Autodesk Inventor part; units mm, degrees
(part 3 of 3)
  line L541 (30.6809, 2.8888) -> (31.1045, 2.7392)
  line L542 (31.1045, 2.7392) -> (31.1501, 2.1604)
  line L543 (31.1501, 2.1604) -> (30.7551, 1.9463)
  line L544 (30.7551, 1.9463) -> (30.3579, 1.7492)
  line L545 (30.3579, 1.7492) -> (29.9589, 1.5701)
  line L546 (29.9589, 1.5701) -> (29.5581, 1.4102)
  line L547 (29.5581, 1.4102) -> (29.1557, 1.2717)
  line L548 (29.1557, 1.2717) -> (28.9539, 1.2113)
  line L549 (28.9539, 1.2113) -> (28.8529, 1.1836)
  line L550 (28.8529, 1.1836) -> (28.7518, 1.1577)
  line L551 (28.7518, 1.1577) -> (28.773, 0.3487)
  line L552 (28.773, 0.3487) -> (28.8753, 0.3281)
  line L553 (28.8753, 0.3281) -> (28.9776, 0.3057)
  line L554 (28.9776, 0.3057) -> (29.1823, 0.256)
  line L555 (29.1823, 0.256) -> (29.5914, 0.1387)
  line L556 (29.5914, 0.1387) -> (30, 0)
  line L557 (30, 0) -> (30.4079, -0.158)
  line L558 (30.4079, -0.158) -> (30.8148, -0.3341)
  line L559 (30.8148, -0.3341) -> (31.2205, -0.5271)
  line L560 (31.2205, -0.5271) -> (31.2053, -1.1075)
  line L561 (31.2053, -1.1075) -> (30.7901, -1.2791)
  line L562 (30.7901, -1.2791) -> (30.3745, -1.4336)
  line L563 (30.3745, -1.4336) -> (29.9589, -1.5701)
  line L564 (29.9589, -1.5701) -> (29.5436, -1.6872)
  line L565 (29.5436, -1.6872) -> (29.1289, -1.7829)
  line L566 (29.1289, -1.7829) -> (28.9219, -1.8218)
  line L567 (28.9219, -1.8218) -> (28.8186, -1.8388)
  line L568 (28.8186, -1.8388) -> (28.7153, -1.854)
  line L569 (28.7153, -1.854) -> (28.6518, -2.6609)
  line L570 (28.6518, -2.6609) -> (28.7514, -2.692)
  line L571 (28.7514, -2.692) -> (28.8508, -2.725)
  line L572 (28.8508, -2.725) -> (29.0492, -2.7958)
  line L573 (29.0492, -2.7958) -> (29.4438, -2.9552)
  line L574 (29.4438, -2.9552) -> (29.8357, -3.1359)
  line L575 (29.8357, -3.1359) -> (30.2248, -3.3356)
  line L576 (30.2248, -3.3356) -> (30.6111, -3.5533)
  line L577 (30.6111, -3.5533) -> (30.9943, -3.7877)
  line L578 (30.9943, -3.7877) -> (30.9185, -4.3633)
  line L579 (30.9185, -4.3633) -> (30.4877, -4.4905)
  line L580 (30.4877, -4.4905) -> (30.0582, -4.6008)
  line L581 (30.0582, -4.6008) -> (29.6307, -4.693)
  line L582 (29.6307, -4.693) -> (29.2054, -4.7661)
  line L583 (29.2054, -4.7661) -> (28.7829, -4.8179)
  line L584 (28.7829, -4.8179) -> (28.5731, -4.835)
  line L585 (28.5731, -4.835) -> (28.4685, -4.8411)
  line L586 (28.4685, -4.8411) -> (28.3642, -4.8455)
  line L587 (28.3642, -4.8455) -> (28.2167, -5.6412)
  line L588 (28.2167, -5.6412) -> (28.3125, -5.6826)
  line L589 (28.3125, -5.6826) -> (28.408, -5.7258)
  line L590 (28.408, -5.7258) -> (28.5978, -5.8169)
  line L591 (28.5978, -5.8169) -> (28.9736, -6.0168)
  line L592 (28.9736, -6.0168) -> (29.3444, -6.2373)
  line L593 (29.3444, -6.2373) -> (29.7106, -6.4767)
  line L594 (29.7106, -6.4767) -> (30.072, -6.7335)
  line L595 (30.072, -6.7335) -> (30.4286, -7.0067)
  line L596 (30.4286, -7.0067) -> (30.2931, -7.5713)
  line L597 (30.2931, -7.5713) -> (29.8513, -7.6528)
  line L598 (29.8513, -7.6528) -> (29.4127, -7.7175)
  line L599 (29.4127, -7.7175) -> (28.9778, -7.7646)
  line L600 (28.9778, -7.7646) -> (28.5472, -7.7927)
  line L601 (28.5472, -7.7927) -> (28.1217, -7.8002)
  line L602 (28.1217, -7.8002) -> (27.9111, -7.7952)
  line L603 (27.9111, -7.7952) -> (27.8065, -7.7904)
  line L604 (27.8065, -7.7904) -> (27.7023, -7.7838)
  line L605 (27.7023, -7.7838) -> (27.4725, -8.5597)
  line L606 (27.4725, -8.5597) -> (27.5634, -8.611)
  line L607 (27.5634, -8.611) -> (27.6538, -8.6638)
  line L608 (27.6538, -8.6638) -> (27.8331, -8.7744)
  line L609 (27.8331, -8.7744) -> (28.1859, -9.0124)
  line L610 (28.1859, -9.0124) -> (28.5317, -9.2705)
  line L611 (28.5317, -9.2705) -> (28.8708, -9.5468)
  line L612 (28.8708, -9.5468) -> (29.2034, -9.84)
  line L613 (29.2034, -9.84) -> (29.5295, -10.149)
  line L614 (29.5295, -10.149) -> (29.3357, -10.6963)
  line L615 (29.3357, -10.6963) -> (28.8878, -10.7312)
  line L616 (28.8878, -10.7312) -> (28.4448, -10.7497)
  line L617 (28.4448, -10.7497) -> (28.0074, -10.751)
  line L618 (28.0074, -10.751) -> (27.5762, -10.7341)
  line L619 (27.5762, -10.7341) -> (27.1523, -10.697)
  line L620 (27.1523, -10.697) -> (26.9434, -10.67)
  line L621 (26.9434, -10.67) -> (26.8398, -10.6543)
  line L622 (26.8398, -10.6543) -> (26.7369, -10.6368)
  line L623 (26.7369, -10.6368) -> (26.4272, -11.3845)
  line L624 (26.4272, -11.3845) -> (26.5123, -11.4449)
  line L625 (26.5123, -11.4449) -> (26.5967, -11.507)
  line L626 (26.5967, -11.507) -> (26.7635, -11.6357)
  line L627 (26.7635, -11.6357) -> (27.0895, -11.9092)
  line L628 (27.0895, -11.9092) -> (27.4064, -12.2021)
  line L629 (27.4064, -12.2021) -> (27.7147, -12.5124)
  line L630 (27.7147, -12.5124) -> (28.0148, -12.8387)
  line L631 (28.0148, -12.8387) -> (28.3069, -13.1801)
  line L632 (28.3069, -13.1801) -> (28.057, -13.7041)
  line L633 (28.057, -13.7041) -> (27.6078, -13.692)
  line L634 (27.6078, -13.692) -> (27.1654, -13.6641)
  line L635 (27.1654, -13.6641) -> (26.7302, -13.6197)
  line L636 (26.7302, -13.6197) -> (26.3032, -13.5578)
  line L637 (26.3032, -13.5578) -> (25.8854, -13.4766)
  line L638 (25.8854, -13.4766) -> (25.6805, -13.4279)
  line L639 (25.6805, -13.4279) -> (25.5791, -13.4014)
  line L640 (25.5791, -13.4014) -> (25.4786, -13.3733)
  line L641 (25.4786, -13.3733) -> (25.0925, -14.0845)
  line L642 (25.0925, -14.0845) -> (25.1708, -14.1535)
  line L643 (25.1708, -14.1535) -> (25.2482, -14.2241)
  line L644 (25.2482, -14.2241) -> (25.4006, -14.3694)
  line L645 (25.4006, -14.3694) -> (25.6962, -14.6756)
  line L646 (25.6962, -14.6756) -> (25.9808, -15)
  line L647 (25.9808, -15) -> (26.255, -15.3408)
  line L648 (26.255, -15.3408) -> (26.5194, -15.6967)
  line L649 (26.5194, -15.6967) -> (26.7741, -16.0667)
  line L650 (26.7741, -16.0667) -> (26.4708, -16.5618)
  line L651 (26.4708, -16.5618) -> (26.0254, -16.5028)
  line L652 (26.0254, -16.5028) -> (25.5883, -16.4288)
  line L653 (25.5883, -16.4288) -> (25.1601, -16.3392)
  line L654 (25.1601, -16.3392) -> (24.7419, -16.2329)
  line L655 (24.7419, -16.2329) -> (24.3349, -16.1085)
  line L656 (24.3349, -16.1085) -> (24.1362, -16.0387)
  line L657 (24.1362, -16.0387) -> (24.0382, -16.0018)
  line L658 (24.0382, -16.0018) -> (23.9412, -15.9633)
  line L659 (23.9412, -15.9633) -> (23.4828, -16.6303)
  line L660 (23.4828, -16.6303) -> (23.5534, -16.7071)
  line L661 (23.5534, -16.7071) -> (23.6231, -16.7853)
  line L662 (23.6231, -16.7853) -> (23.7594, -16.9458)
  line L663 (23.7594, -16.9458) -> (24.0214, -17.2812)
  line L664 (24.0214, -17.2812) -> (24.2705, -17.6336)
  line L665 (24.2705, -17.6336) -> (24.5076, -18.0012)
  line L666 (24.5076, -18.0012) -> (24.7333, -18.3827)
  line L667 (24.7333, -18.3827) -> (24.948, -18.7774)
  line L668 (24.948, -18.7774) -> (24.5946, -19.238)
  line L669 (24.5946, -19.238) -> (24.1578, -19.1328)
  line L670 (24.1578, -19.1328) -> (23.7308, -19.0135)
  line L671 (23.7308, -19.0135) -> (23.3144, -18.8796)
  line L672 (23.3144, -18.8796) -> (22.9095, -18.7302)
  line L673 (22.9095, -18.7302) -> (22.5178, -18.5639)
  line L674 (22.5178, -18.5639) -> (22.3275, -18.4738)
  line L675 (22.3275, -18.4738) -> (22.2339, -18.4268)
  line L676 (22.2339, -18.4268) -> (22.1414, -18.3784)
  line L677 (22.1414, -18.3784) -> (21.6158, -18.9938)
  line L678 (21.6158, -18.9938) -> (21.6781, -19.0775)
  line L679 (21.6781, -19.0775) -> (21.7391, -19.1626)
  line L680 (21.7391, -19.1626) -> (21.8579, -19.3365)
  line L681 (21.8579, -19.3365) -> (22.0835, -19.6974)
  line L682 (22.0835, -19.6974) -> (22.2943, -20.0739)
  line L683 (22.2943, -20.0739) -> (22.4917, -20.4643)
  line L684 (22.4917, -20.4643) -> (22.6763, -20.8674)
  line L685 (22.6763, -20.8674) -> (22.8486, -21.2823)
  line L686 (22.8486, -21.2823) -> (22.4489, -21.7034)
  line L687 (22.4489, -21.7034) -> (22.0256, -21.5531)
  line L688 (22.0256, -21.5531) -> (21.6134, -21.3899)
  line L689 (21.6134, -21.3899) -> (21.2132, -21.2132)
  line L690 (21.2132, -21.2132) -> (20.8262, -21.0223)
  line L691 (20.8262, -21.0223) -> (20.454, -20.816)
  line L692 (20.454, -20.816) -> (20.2741, -20.7064)
  line L693 (20.2741, -20.7064) -> (20.1859, -20.6499)
  line L694 (20.1859, -20.6499) -> (20.099, -20.5921)
  line L695 (20.099, -20.5921) -> (19.512, -21.1492)
  line L696 (19.512, -21.1492) -> (19.5652, -21.239)
  line L697 (19.5652, -21.239) -> (19.617, -21.33)
  line L698 (19.617, -21.33) -> (19.717, -21.5154)
  line L699 (19.717, -21.5154) -> (19.9035, -21.8979)
  line L700 (19.9035, -21.8979) -> (20.0739, -22.2943)
  line L701 (20.0739, -22.2943) -> (20.2294, -22.7032)
  line L702 (20.2294, -22.7032) -> (20.3709, -23.1234)
  line L703 (20.3709, -23.1234) -> (20.4988, -23.5541)
  line L704 (20.4988, -23.5541) -> (20.0573, -23.9311)
  line L705 (20.0573, -23.9311) -> (19.652, -23.7374)
  line L706 (19.652, -23.7374) -> (19.2591, -23.5319)
  line L707 (19.2591, -23.5319) -> (18.8796, -23.3144)
  line L708 (18.8796, -23.3144) -> (18.5147, -23.0841)
  line L709 (18.5147, -23.0841) -> (18.1661, -22.84)
  line L710 (18.1661, -22.84) -> (17.9986, -22.7122)
  line L711 (17.9986, -22.7122) -> (17.9169, -22.6468)
  line L712 (17.9169, -22.6468) -> (17.8365, -22.5802)
  line L713 (17.8365, -22.5802) -> (17.1944, -23.0729)
  line L714 (17.1944, -23.0729) -> (17.2379, -23.1678)
  line L715 (17.2379, -23.1678) -> (17.2799, -23.2637)
  line L716 (17.2799, -23.2637) -> (17.36, -23.4585)
  line L717 (17.36, -23.4585) -> (17.5056, -23.8584)
  line L718 (17.5056, -23.8584) -> (17.6336, -24.2705)
  line L719 (17.6336, -24.2705) -> (17.7455, -24.6934)
  line L720 (17.7455, -24.6934) -> (17.8422, -25.1261)
  line L721 (17.8422, -25.1261) -> (17.9245, -25.5677)
  line L722 (17.9245, -25.5677) -> (17.446, -25.8966)
  line L723 (17.446, -25.8966) -> (17.0631, -25.6615)
  line L724 (17.0631, -25.6615) -> (16.6939, -25.4161)
  line L725 (16.6939, -25.4161) -> (16.3392, -25.1601)
  line L726 (16.3392, -25.1601) -> (16.0003, -24.8929)
  line L727 (16.0003, -24.8929) -> (15.6791, -24.6137)
  line L728 (15.6791, -24.6137) -> (15.526, -24.4692)
  line L729 (15.526, -24.4692) -> (15.4515, -24.3955)
  line L730 (15.4515, -24.3955) -> (15.3785, -24.3209)
  line L731 (15.3785, -24.3209) -> (14.6884, -24.7438)
  line L732 (14.6884, -24.7438) -> (14.7218, -24.8427)
  line L733 (14.7218, -24.8427) -> (14.7536, -24.9425)
  line L734 (14.7536, -24.9425) -> (14.8128, -25.1446)
  line L735 (14.8128, -25.1446) -> (14.9158, -25.5575)
  line L736 (14.9158, -25.5575) -> (15, -25.9808)
  line L737 (15, -25.9808) -> (15.0671, -26.413)
  line L738 (15.0671, -26.413) -> (15.1181, -26.8534)
  line L739 (15.1181, -26.8534) -> (15.1537, -27.3013)
  line L740 (15.1537, -27.3013) -> (14.6435, -27.5783)
  line L741 (14.6435, -27.5783) -> (14.2873, -27.3045)
  line L742 (14.2873, -27.3045) -> (13.9457, -27.0219)
  line L743 (13.9457, -27.0219) -> (13.6197, -26.7302)
  line L744 (13.6197, -26.7302) -> (13.3107, -26.4291)
  line L745 (13.3107, -26.4291) -> (13.0204, -26.1178)
  line L746 (13.0204, -26.1178) -> (12.8832, -25.958)
  line L747 (12.8832, -25.958) -> (12.8168, -25.877)
  line L748 (12.8168, -25.877) -> (12.752, -25.7952)
  line L749 (12.752, -25.7952) -> (12.0215, -26.1436)
  line L750 (12.0215, -26.1436) -> (12.0443, -26.2455)
  line L751 (12.0443, -26.2455) -> (12.0655, -26.348)
  line L752 (12.0655, -26.348) -> (12.1033, -26.5552)
  line L753 (12.1033, -26.5552) -> (12.1626, -26.9767)
  line L754 (12.1626, -26.9767) -> (12.2021, -27.4064)
  line L755 (12.2021, -27.4064) -> (12.2236, -27.8433)
  line L756 (12.2236, -27.8433) -> (12.2283, -28.2866)
  line L757 (12.2283, -28.2866) -> (12.2169, -28.7357)
  line L758 (12.2169, -28.7357) -> (11.6805, -28.9579)
  line L759 (11.6805, -28.9579) -> (11.3549, -28.6484)
  line L760 (11.3549, -28.6484) -> (11.0447, -28.3316)
  line L761 (11.0447, -28.3316) -> (10.751, -28.0074)
  line L762 (10.751, -28.0074) -> (10.4751, -27.6756)
  line L763 (10.4751, -27.6756) -> (10.219, -27.3357)
  line L764 (10.219, -27.3357) -> (10.0993, -27.1625)
  line L765 (10.0993, -27.1625) -> (10.0417, -27.075)
  line L766 (10.0417, -27.075) -> (9.9858, -26.9868)
  line L767 (9.9858, -26.9868) -> (9.2229, -27.257)
  line L768 (9.2229, -27.257) -> (9.235, -27.3607)
  line L769 (9.235, -27.3607) -> (9.2453, -27.4649)
  line L770 (9.2453, -27.4649) -> (9.2613, -27.6749)
  line L771 (9.2613, -27.6749) -> (9.2761, -28.1002)
  line L772 (9.2761, -28.1002) -> (9.2705, -28.5317)
  line L773 (9.2705, -28.5317) -> (9.2463, -28.9685)
  line L774 (9.2463, -28.9685) -> (9.2046, -29.4098)
  line L775 (9.2046, -29.4098) -> (9.1463, -29.8553)
  line L776 (9.1463, -29.8553) -> (8.5896, -30.0202)
  line L777 (8.5896, -30.0202) -> (8.2981, -29.6783)
  line L778 (8.2981, -29.6783) -> (8.0228, -29.3309)
  line L779 (8.0228, -29.3309) -> (7.7646, -28.9778)
  line L780 (7.7646, -28.9778) -> (7.5249, -28.619)
  line L781 (7.5249, -28.619) -> (7.3057, -28.2542)
  line L782 (7.3057, -28.2542) -> (7.2047, -28.0694)
  line L783 (7.2047, -28.0694) -> (7.1566, -27.9763)
  line L784 (7.1566, -27.9763) -> (7.1102, -27.8828)
  line L785 (7.1102, -27.8828) -> (6.3233, -28.0717)
  line L786 (6.3233, -28.0717) -> (6.3244, -28.1761)
  line L787 (6.3244, -28.1761) -> (6.3238, -28.2808)
  line L788 (6.3238, -28.2808) -> (6.3177, -28.4913)
  line L789 (6.3177, -28.4913) -> (6.288, -28.9159)
  line L790 (6.288, -28.9159) -> (6.2374, -29.3444)
  line L791 (6.2374, -29.3444) -> (6.1676, -29.7763)
  line L792 (6.1676, -29.7763) -> (6.08, -30.2109)
  line L793 (6.08, -30.2109) -> (5.9755, -30.6478)
  line L794 (5.9755, -30.6478) -> (5.4046, -30.7536)
  line L795 (5.4046, -30.7536) -> (5.1505, -30.3831)
  line L796 (5.1505, -30.3831) -> (4.9129, -30.0088)
  line L797 (4.9129, -30.0088) -> (4.693, -29.6306)
  line L798 (4.693, -29.6306) -> (4.4922, -29.2487)
  line L799 (4.4922, -29.2487) -> (4.3123, -28.863)
  line L800 (4.3123, -28.863) -> (4.2312, -28.6687)
  line L801 (4.2312, -28.6687) -> (4.1931, -28.5711)
  line L802 (4.1931, -28.5711) -> (4.1567, -28.4733)
  line L803 (4.1567, -28.4733) -> (3.3543, -28.5789)
  line L804 (3.3543, -28.5789) -> (3.3446, -28.6828)
  line L805 (3.3446, -28.6828) -> (3.333, -28.7869)
  line L806 (3.333, -28.7869) -> (3.305, -28.9957)
  line L807 (3.305, -28.9957) -> (3.231, -29.4148)
  line L808 (3.231, -29.4148) -> (3.1359, -29.8357)
  line L809 (3.1359, -29.8357) -> (3.0213, -30.2578)
  line L810 (3.0213, -30.2578) -> (2.8888, -30.6809)
  line L811 (2.8888, -30.6809) -> (2.7392, -31.1045)
  line L812 (2.7392, -31.1045) -> (2.1604, -31.1501)
  line L813 (2.1604, -31.1501) -> (1.9463, -30.7551)
  line L814 (1.9463, -30.7551) -> (1.7492, -30.3579)
  line L815 (1.7492, -30.3579) -> (1.5701, -29.9589)
  line L816 (1.5701, -29.9589) -> (1.4102, -29.5581)
  line L817 (1.4102, -29.5581) -> (1.2717, -29.1557)
  line L818 (1.2717, -29.1557) -> (1.2113, -28.9539)
  line L819 (1.2113, -28.9539) -> (1.1836, -28.8529)
  line L820 (1.1836, -28.8529) -> (1.1577, -28.7518)
  line L821 (1.1577, -28.7518) -> (0.3487, -28.773)
  line L822 (0.3487, -28.773) -> (0.3281, -28.8753)
  line L823 (0.3281, -28.8753) -> (0.3057, -28.9776)
  line L824 (0.3057, -28.9776) -> (0.256, -29.1823)
  line L825 (0.256, -29.1823) -> (0.1387, -29.5914)
  line L826 (0.1387, -29.5914) -> (0, -30)
  line L827 (0, -30) -> (-0.158, -30.4079)
  line L828 (-0.158, -30.4079) -> (-0.3341, -30.8148)
  line L829 (-0.3341, -30.8148) -> (-0.5272, -31.2205)
  line L830 (-0.5272, -31.2205) -> (-1.1075, -31.2053)
  line L831 (-1.1075, -31.2053) -> (-1.2791, -30.79)
  line L832 (-1.2791, -30.79) -> (-1.4336, -30.3745)
  line L833 (-1.4336, -30.3745) -> (-1.5701, -29.9589)
  line L834 (-1.5701, -29.9589) -> (-1.6872, -29.5436)
  line L835 (-1.6872, -29.5436) -> (-1.7829, -29.1289)
  line L836 (-1.7829, -29.1289) -> (-1.8218, -28.9219)
  line L837 (-1.8218, -28.9219) -> (-1.8388, -28.8186)
  line L838 (-1.8388, -28.8186) -> (-1.854, -28.7153)
  line L839 (-1.854, -28.7153) -> (-2.6609, -28.6518)
  line L840 (-2.6609, -28.6518) -> (-2.692, -28.7514)
  line L841 (-2.692, -28.7514) -> (-2.725, -28.8508)
  line L842 (-2.725, -28.8508) -> (-2.7958, -29.0492)
  line L843 (-2.7958, -29.0492) -> (-2.9552, -29.4438)
  line L844 (-2.9552, -29.4438) -> (-3.1359, -29.8357)
  line L845 (-3.1359, -29.8357) -> (-3.3357, -30.2248)
  line L846 (-3.3357, -30.2248) -> (-3.5533, -30.6111)
  line L847 (-3.5533, -30.6111) -> (-3.7877, -30.9943)
  line L848 (-3.7877, -30.9943) -> (-4.3633, -30.9185)
  line L849 (-4.3633, -30.9185) -> (-4.4905, -30.4877)
  line L850 (-4.4905, -30.4877) -> (-4.6008, -30.0582)
  line L851 (-4.6008, -30.0582) -> (-4.693, -29.6306)
  line L852 (-4.693, -29.6306) -> (-4.7661, -29.2054)
  line L853 (-4.7661, -29.2054) -> (-4.8179, -28.7829)
  line L854 (-4.8179, -28.7829) -> (-4.835, -28.573)
  line L855 (-4.835, -28.573) -> (-4.8411, -28.4685)
  line L856 (-4.8411, -28.4685) -> (-4.8455, -28.3642)
  line L857 (-4.8455, -28.3642) -> (-5.6412, -28.2167)
  line L858 (-5.6412, -28.2167) -> (-5.6826, -28.3125)
  line L859 (-5.6826, -28.3125) -> (-5.7258, -28.408)
  line L860 (-5.7258, -28.408) -> (-5.8169, -28.5978)
  line L861 (-5.8169, -28.5978) -> (-6.0168, -28.9736)
  line L862 (-6.0168, -28.9736) -> (-6.2374, -29.3444)
  line L863 (-6.2374, -29.3444) -> (-6.4767, -29.7105)
  line L864 (-6.4767, -29.7105) -> (-6.7335, -30.072)
  line L865 (-6.7335, -30.072) -> (-7.0067, -30.4286)
  line L866 (-7.0067, -30.4286) -> (-7.5713, -30.2931)
  line L867 (-7.5713, -30.2931) -> (-7.6528, -29.8513)
  line L868 (-7.6528, -29.8513) -> (-7.7175, -29.4127)
  line L869 (-7.7175, -29.4127) -> (-7.7646, -28.9778)
  line L870 (-7.7646, -28.9778) -> (-7.7927, -28.5472)
  line L871 (-7.7927, -28.5472) -> (-7.8002, -28.1217)
  line L872 (-7.8002, -28.1217) -> (-7.7952, -27.9111)
  line L873 (-7.7952, -27.9111) -> (-7.7904, -27.8065)
  line L874 (-7.7904, -27.8065) -> (-7.7838, -27.7023)
  line L875 (-7.7838, -27.7023) -> (-8.5597, -27.4725)
  line L876 (-8.5597, -27.4725) -> (-8.611, -27.5634)
  line L877 (-8.611, -27.5634) -> (-8.6638, -27.6538)
  line L878 (-8.6638, -27.6538) -> (-8.7744, -27.8331)
  line L879 (-8.7744, -27.8331) -> (-9.0124, -28.1859)
  line L880 (-9.0124, -28.1859) -> (-9.2705, -28.5317)
  line L881 (-9.2705, -28.5317) -> (-9.5468, -28.8708)
  line L882 (-9.5468, -28.8708) -> (-9.84, -29.2034)
  line L883 (-9.84, -29.2034) -> (-10.149, -29.5295)
  line L884 (-10.149, -29.5295) -> (-10.6963, -29.3357)
  line L885 (-10.6963, -29.3357) -> (-10.7312, -28.8878)
  line L886 (-10.7312, -28.8878) -> (-10.7497, -28.4448)
  line L887 (-10.7497, -28.4448) -> (-10.751, -28.0074)
  line L888 (-10.751, -28.0074) -> (-10.7341, -27.5762)
  line L889 (-10.7341, -27.5762) -> (-10.697, -27.1523)
  line L890 (-10.697, -27.1523) -> (-10.67, -26.9434)
  line L891 (-10.67, -26.9434) -> (-10.6543, -26.8398)
  line L892 (-10.6543, -26.8398) -> (-10.6368, -26.7369)
  line L893 (-10.6368, -26.7369) -> (-11.3845, -26.4272)
  line L894 (-11.3845, -26.4272) -> (-11.4449, -26.5123)
  line L895 (-11.4449, -26.5123) -> (-11.507, -26.5967)
  line L896 (-11.507, -26.5967) -> (-11.6357, -26.7634)
  line L897 (-11.6357, -26.7634) -> (-11.9092, -27.0895)
  line L898 (-11.9092, -27.0895) -> (-12.2021, -27.4064)
  line L899 (-12.2021, -27.4064) -> (-12.5124, -27.7147)
  line L900 (-12.5124, -27.7147) -> (-12.8387, -28.0148)
  line L901 (-12.8387, -28.0148) -> (-13.1801, -28.3069)
  line L902 (-13.1801, -28.3069) -> (-13.7041, -28.0569)
  line L903 (-13.7041, -28.0569) -> (-13.692, -27.6078)
  line L904 (-13.692, -27.6078) -> (-13.6641, -27.1654)
  line L905 (-13.6641, -27.1654) -> (-13.6197, -26.7302)
  line L906 (-13.6197, -26.7302) -> (-13.5578, -26.3031)
  line L907 (-13.5578, -26.3031) -> (-13.4766, -25.8854)
  line L908 (-13.4766, -25.8854) -> (-13.4279, -25.6805)
  line L909 (-13.4279, -25.6805) -> (-13.4014, -25.5791)
  line L910 (-13.4014, -25.5791) -> (-13.3733, -25.4786)
  line L911 (-13.3733, -25.4786) -> (-14.0845, -25.0925)
  line L912 (-14.0845, -25.0925) -> (-14.1535, -25.1708)
  line L913 (-14.1535, -25.1708) -> (-14.2241, -25.2482)
  line L914 (-14.2241, -25.2482) -> (-14.3694, -25.4006)
  line L915 (-14.3694, -25.4006) -> (-14.6756, -25.6962)
  line L916 (-14.6756, -25.6962) -> (-15, -25.9808)
  line L917 (-15, -25.9808) -> (-15.3408, -26.255)
  line L918 (-15.3408, -26.255) -> (-15.6967, -26.5194)
  line L919 (-15.6967, -26.5194) -> (-16.0668, -26.7741)
  line L920 (-16.0668, -26.7741) -> (-16.5618, -26.4708)
  line L921 (-16.5618, -26.4708) -> (-16.5028, -26.0254)
  line L922 (-16.5028, -26.0254) -> (-16.4288, -25.5883)
  line L923 (-16.4288, -25.5883) -> (-16.3392, -25.1601)
  line L924 (-16.3392, -25.1601) -> (-16.2329, -24.7419)
  line L925 (-16.2329, -24.7419) -> (-16.1085, -24.3349)
  line L926 (-16.1085, -24.3349) -> (-16.0387, -24.1362)
  line L927 (-16.0387, -24.1362) -> (-16.0018, -24.0382)
  line L928 (-16.0018, -24.0382) -> (-15.9633, -23.9412)
  line L929 (-15.9633, -23.9412) -> (-16.6303, -23.4828)
  line L930 (-16.6303, -23.4828) -> (-16.7071, -23.5534)
  line L931 (-16.7071, -23.5534) -> (-16.7853, -23.6231)
  line L932 (-16.7853, -23.6231) -> (-16.9458, -23.7594)
  line L933 (-16.9458, -23.7594) -> (-17.2812, -24.0214)
  line L934 (-17.2812, -24.0214) -> (-17.6336, -24.2705)
  line L935 (-17.6336, -24.2705) -> (-18.0012, -24.5076)
  line L936 (-18.0012, -24.5076) -> (-18.3827, -24.7333)
  line L937 (-18.3827, -24.7333) -> (-18.7774, -24.948)
  line L938 (-18.7774, -24.948) -> (-19.238, -24.5946)
  line L939 (-19.238, -24.5946) -> (-19.1328, -24.1578)
  line L940 (-19.1328, -24.1578) -> (-19.0135, -23.7308)
  line L941 (-19.0135, -23.7308) -> (-18.8796, -23.3144)
  line L942 (-18.8796, -23.3144) -> (-18.7302, -22.9096)
  line L943 (-18.7302, -22.9096) -> (-18.5639, -22.5178)
  line L944 (-18.5639, -22.5178) -> (-18.4738, -22.3275)
  line L945 (-18.4738, -22.3275) -> (-18.4268, -22.2339)
  line L946 (-18.4268, -22.2339) -> (-18.3784, -22.1414)
  line L947 (-18.3784, -22.1414) -> (-18.9938, -21.6158)
  line L948 (-18.9938, -21.6158) -> (-19.0775, -21.6781)
  line L949 (-19.0775, -21.6781) -> (-19.1627, -21.7391)
  line L950 (-19.1627, -21.7391) -> (-19.3365, -21.8579)
  line L951 (-19.3365, -21.8579) -> (-19.6974, -22.0835)
  line L952 (-19.6974, -22.0835) -> (-20.0739, -22.2943)
  line L953 (-20.0739, -22.2943) -> (-20.4643, -22.4917)
  line L954 (-20.4643, -22.4917) -> (-20.8674, -22.6763)
  line L955 (-20.8674, -22.6763) -> (-21.2823, -22.8486)
  line L956 (-21.2823, -22.8486) -> (-21.7034, -22.4489)
  line L957 (-21.7034, -22.4489) -> (-21.5531, -22.0256)
  line L958 (-21.5531, -22.0256) -> (-21.3899, -21.6134)
  line L959 (-21.3899, -21.6134) -> (-21.2132, -21.2132)
  line L960 (-21.2132, -21.2132) -> (-21.0223, -20.8262)
  line L961 (-21.0223, -20.8262) -> (-20.816, -20.454)
  line L962 (-20.816, -20.454) -> (-20.7064, -20.2741)
  line L963 (-20.7064, -20.2741) -> (-20.6499, -20.1859)
  line L964 (-20.6499, -20.1859) -> (-20.5921, -20.099)
  line L965 (-20.5921, -20.099) -> (-21.1492, -19.512)
  line L966 (-21.1492, -19.512) -> (-21.239, -19.5652)
  line L967 (-21.239, -19.5652) -> (-21.33, -19.617)
  line L968 (-21.33, -19.617) -> (-21.5154, -19.717)
  line L969 (-21.5154, -19.717) -> (-21.8979, -19.9035)
  line L970 (-21.8979, -19.9035) -> (-22.2943, -20.0739)
  line L971 (-22.2943, -20.0739) -> (-22.7032, -20.2294)
  line L972 (-22.7032, -20.2294) -> (-23.1234, -20.3709)
  line L973 (-23.1234, -20.3709) -> (-23.5541, -20.4988)
  line L974 (-23.5541, -20.4988) -> (-23.9311, -20.0573)
  line L975 (-23.9311, -20.0573) -> (-23.7374, -19.652)
  line L976 (-23.7374, -19.652) -> (-23.5319, -19.2591)
  line L977 (-23.5319, -19.2591) -> (-23.3144, -18.8796)
  line L978 (-23.3144, -18.8796) -> (-23.0841, -18.5147)
  line L979 (-23.0841, -18.5147) -> (-22.84, -18.1661)
  line L980 (-22.84, -18.1661) -> (-22.7122, -17.9986)
  line L981 (-22.7122, -17.9986) -> (-22.6468, -17.9169)
  line L982 (-22.6468, -17.9169) -> (-22.5802, -17.8365)
  line L983 (-22.5802, -17.8365) -> (-23.0729, -17.1944)
  line L984 (-23.0729, -17.1944) -> (-23.1678, -17.2379)
  line L985 (-23.1678, -17.2379) -> (-23.2637, -17.2799)
  line L986 (-23.2637, -17.2799) -> (-23.4585, -17.36)
  line L987 (-23.4585, -17.36) -> (-23.8584, -17.5055)
  line L988 (-23.8584, -17.5055) -> (-24.2705, -17.6336)
  line L989 (-24.2705, -17.6336) -> (-24.6934, -17.7455)
  line L990 (-24.6934, -17.7455) -> (-25.1261, -17.8422)
  line L991 (-25.1261, -17.8422) -> (-25.5677, -17.9244)
  line L992 (-25.5677, -17.9244) -> (-25.8966, -17.446)
  line L993 (-25.8966, -17.446) -> (-25.6615, -17.0631)
  line L994 (-25.6615, -17.0631) -> (-25.4161, -16.6939)
  line L995 (-25.4161, -16.6939) -> (-25.1601, -16.3392)
  line L996 (-25.1601, -16.3392) -> (-24.8929, -16.0003)
  line L997 (-24.8929, -16.0003) -> (-24.6137, -15.6791)
  line L998 (-24.6137, -15.6791) -> (-24.4692, -15.526)
  line L999 (-24.4692, -15.526) -> (-24.3955, -15.4515)
  line L1000 (-24.3955, -15.4515) -> (-24.3209, -15.3785)
  line L1001 (-24.3209, -15.3785) -> (-24.7438, -14.6884)
  line L1002 (-24.7438, -14.6884) -> (-24.8427, -14.7218)
  line L1003 (-24.8427, -14.7218) -> (-24.9425, -14.7535)
  line L1004 (-24.9425, -14.7535) -> (-25.1446, -14.8128)
  line L1005 (-25.1446, -14.8128) -> (-25.5576, -14.9158)
  line L1006 (-25.5576, -14.9158) -> (-25.9808, -15)
  line L1007 (-25.9808, -15) -> (-26.413, -15.0671)
  line L1008 (-26.413, -15.0671) -> (-26.8534, -15.1181)
  line L1009 (-26.8534, -15.1181) -> (-27.3013, -15.1537)
  line L1010 (-27.3013, -15.1537) -> (-27.5783, -14.6435)
  line L1011 (-27.5783, -14.6435) -> (-27.3045, -14.2873)
  line L1012 (-27.3045, -14.2873) -> (-27.0219, -13.9457)
  line L1013 (-27.0219, -13.9457) -> (-26.7302, -13.6197)
  line L1014 (-26.7302, -13.6197) -> (-26.4291, -13.3106)
  line L1015 (-26.4291, -13.3106) -> (-26.1178, -13.0204)
  line L1016 (-26.1178, -13.0204) -> (-25.958, -12.8832)
  line L1017 (-25.958, -12.8832) -> (-25.877, -12.8168)
  line L1018 (-25.877, -12.8168) -> (-25.7952, -12.752)
  line L1019 (-25.7952, -12.752) -> (-26.1436, -12.0215)
  line L1020 (-26.1436, -12.0215) -> (-26.2455, -12.0443)
  line L1021 (-26.2455, -12.0443) -> (-26.348, -12.0655)
  line L1022 (-26.348, -12.0655) -> (-26.5552, -12.1033)
  line L1023 (-26.5552, -12.1033) -> (-26.9767, -12.1626)
  line L1024 (-26.9767, -12.1626) -> (-27.4064, -12.2021)
  line L1025 (-27.4064, -12.2021) -> (-27.8433, -12.2236)
  line L1026 (-27.8433, -12.2236) -> (-28.2866, -12.2283)
  line L1027 (-28.2866, -12.2283) -> (-28.7357, -12.2169)
  line L1028 (-28.7357, -12.2169) -> (-28.9579, -11.6805)
  line L1029 (-28.9579, -11.6805) -> (-28.6484, -11.3549)
  line L1030 (-28.6484, -11.3549) -> (-28.3316, -11.0447)
  line L1031 (-28.3316, -11.0447) -> (-28.0074, -10.751)
  line L1032 (-28.0074, -10.751) -> (-27.6756, -10.4751)
  line L1033 (-27.6756, -10.4751) -> (-27.3357, -10.219)
  line L1034 (-27.3357, -10.219) -> (-27.1625, -10.0993)
  line L1035 (-27.1625, -10.0993) -> (-27.075, -10.0417)
  line L1036 (-27.075, -10.0417) -> (-26.9868, -9.9858)
  line L1037 (-26.9868, -9.9858) -> (-27.257, -9.2229)
  line L1038 (-27.257, -9.2229) -> (-27.3607, -9.235)
  line L1039 (-27.3607, -9.235) -> (-27.4649, -9.2453)
  line L1040 (-27.4649, -9.2453) -> (-27.6749, -9.2613)
  line L1041 (-27.6749, -9.2613) -> (-28.1002, -9.2761)
  line L1042 (-28.1002, -9.2761) -> (-28.5317, -9.2705)
  line L1043 (-28.5317, -9.2705) -> (-28.9685, -9.2463)
  line L1044 (-28.9685, -9.2463) -> (-29.4098, -9.2046)
  line L1045 (-29.4098, -9.2046) -> (-29.8553, -9.1463)
  line L1046 (-29.8553, -9.1463) -> (-30.0202, -8.5896)
  line L1047 (-30.0202, -8.5896) -> (-29.6783, -8.2981)
  line L1048 (-29.6783, -8.2981) -> (-29.3309, -8.0228)
  line L1049 (-29.3309, -8.0228) -> (-28.9778, -7.7646)
  line L1050 (-28.9778, -7.7646) -> (-28.619, -7.5249)
  line L1051 (-28.619, -7.5249) -> (-28.2542, -7.3057)
  line L1052 (-28.2542, -7.3057) -> (-28.0694, -7.2047)
  line L1053 (-28.0694, -7.2047) -> (-27.9763, -7.1566)
  line L1054 (-27.9763, -7.1566) -> (-27.8828, -7.1102)
  line L1055 (-27.8828, -7.1102) -> (-28.0717, -6.3233)
  line L1056 (-28.0717, -6.3233) -> (-28.1761, -6.3244)
  line L1057 (-28.1761, -6.3244) -> (-28.2808, -6.3238)
  line L1058 (-28.2808, -6.3238) -> (-28.4913, -6.3177)
  line L1059 (-28.4913, -6.3177) -> (-28.9159, -6.288)
  line L1060 (-28.9159, -6.288) -> (-29.3444, -6.2373)
  line L1061 (-29.3444, -6.2373) -> (-29.7763, -6.1676)
  line L1062 (-29.7763, -6.1676) -> (-30.2109, -6.08)
  line L1063 (-30.2109, -6.08) -> (-30.6478, -5.9755)
  line L1064 (-30.6478, -5.9755) -> (-30.7536, -5.4046)
  line L1065 (-30.7536, -5.4046) -> (-30.3831, -5.1504)
  line L1066 (-30.3831, -5.1504) -> (-30.0088, -4.9129)
  line L1067 (-30.0088, -4.9129) -> (-29.6306, -4.693)
  line L1068 (-29.6306, -4.693) -> (-29.2487, -4.4922)
  line L1069 (-29.2487, -4.4922) -> (-28.863, -4.3123)
  line L1070 (-28.863, -4.3123) -> (-28.6687, -4.2312)
  line L1071 (-28.6687, -4.2312) -> (-28.5711, -4.1931)
  line L1072 (-28.5711, -4.1931) -> (-28.4733, -4.1567)
  line L1073 (-28.4733, -4.1567) -> (-28.5789, -3.3543)
  line L1074 (-28.5789, -3.3543) -> (-28.6828, -3.3446)
  line L1075 (-28.6828, -3.3446) -> (-28.7869, -3.333)
  line L1076 (-28.7869, -3.333) -> (-28.9957, -3.3049)
  line L1077 (-28.9957, -3.3049) -> (-29.4148, -3.231)
  line L1078 (-29.4148, -3.231) -> (-29.8357, -3.1359)
  line L1079 (-29.8357, -3.1359) -> (-30.2578, -3.0213)
  line L1080 (-30.2578, -3.0213) -> (-30.6809, -2.8888)
  line L1081 (-30.6809, -2.8888) -> (-31.1045, -2.7392)
  line L1082 (-31.1045, -2.7392) -> (-31.1501, -2.1604)
  line L1083 (-31.1501, -2.1604) -> (-30.7551, -1.9463)
  line L1084 (-30.7551, -1.9463) -> (-30.3579, -1.7492)
  line L1085 (-30.3579, -1.7492) -> (-29.9589, -1.5701)
  line L1086 (-29.9589, -1.5701) -> (-29.5581, -1.4102)
  line L1087 (-29.5581, -1.4102) -> (-29.1557, -1.2716)
  line L1088 (-29.1557, -1.2716) -> (-28.9539, -1.2113)
  line L1089 (-28.9539, -1.2113) -> (-28.8529, -1.1836)
  line L1090 (-28.8529, -1.1836) -> (-28.7518, -1.1577)
  line L1091 (-28.7518, -1.1577) -> (-28.773, -0.3487)
  line L1092 (-28.773, -0.3487) -> (-28.8753, -0.3281)
  line L1093 (-28.8753, -0.3281) -> (-28.9776, -0.3057)
  line L1094 (-28.9776, -0.3057) -> (-29.1823, -0.256)
  line L1095 (-29.1823, -0.256) -> (-29.5914, -0.1387)
  line L1096 (-29.5914, -0.1387) -> (-30, 0)
  line L1097 (-30, 0) -> (-30.4079, 0.158)
  line L1098 (-30.4079, 0.158) -> (-30.8148, 0.3341)
  line L1099 (-30.8148, 0.3341) -> (-31.2205, 0.5271)
  line L1100 (-31.2205, 0.5271) -> (-31.2053, 1.1075)
  line L1101 (-31.2053, 1.1075) -> (-30.79, 1.2791)
  line L1102 (-30.79, 1.2791) -> (-30.3745, 1.4336)
  line L1103 (-30.3745, 1.4336) -> (-29.9589, 1.5701)
  line L1104 (-29.9589, 1.5701) -> (-29.5436, 1.6872)
  line L1105 (-29.5436, 1.6872) -> (-29.1289, 1.7829)
  line L1106 (-29.1289, 1.7829) -> (-28.9219, 1.8218)
  line L1107 (-28.9219, 1.8218) -> (-28.8186, 1.8388)
  line L1108 (-28.8186, 1.8388) -> (-28.7153, 1.854)
  line L1109 (-28.7153, 1.854) -> (-28.6518, 2.6609)
  circle A43 centre (0, 0) radius 0.5
  line L1110 (31.2129, -0.8173) -> (-31.2129, 0.8173) construction
  point P0 (15.2561, 7.5)
  point P1 (7.5, 15.2561)
  point P2 (0, 0)
  point P3 (24.6568, 7.5)
  point P4 (7.5, 24.6568)
  point P5 (0, 0)
  point P6 (-15.2561, 7.5)
  point P7 (-7.5, 15.2561)
  point P8 (-7.5, -15.2561)
  point P9 (-15.2561, -7.5)
  point P10 (15.2561, -7.5)
  point P11 (7.5, -15.2561)
  dimension "d18" = 1
  dimension "d21" = 360
  dimension "d23" = 2
  dimension "d24" = 2
  dimension "d25" = 2
  dimension "d26" = 2
  dimension "d27" = 2
  dimension "d30" = 360
  dimension "d40" = 1.5
  constraints: 99 point on circle, 52 end point, 42 centre point, 11 point on line, 8 tangent, 6 coincident, 5 equal radius, 4 collinear, 2 parallel, 1 vertical, 179 other
  measures "d23" radial gap between concentric circles of A1 A19
  measures "d24" distance between parallel lines of L21 L20
  measures "d25" distance between parallel lines of L22 L1
  measures "d26" radial gap between concentric circles of A3 A20
  measures "d27" radius of A21
  measures "d40" angle of L0 L29
extrude "Extrusion9" add sketch "Sketch7" along normal mid plane 1 contours L2 A1 L7 A0 | A3 L20 A1 L1 | L8 A1 L9 A3 | A3 L18 A1 L19 | L10 A1 L11 A3 | A3 L16 A1 L17 | L12 A1 L13 A3 | A3 L14 A1 L15
extrude "Extrusion11" add sketch "Sketch7" along normal mid plane 5 contours A2 L1 A1 L2 | L7 A1 L8 A4 | A3 L19 A1 L20 | L9 A1 L10 A3 | A3 L17 A1 L18 | L11 A1 L12 A3 | A3 L15 A1 L16 | L13 A1 L14 A3
extrude "Extrusion12" add sketch "Sketch7" along normal mid plane 5 contours L30 L31 L32 L33 L34 L35 L36 L37 L38 L39 L40 L41 L42 L43 L44 L45 L46 L47 L48 L49 L50 L51 L52 L53 L54 L55 L56 L57 L58 L59 L60 L61 L62 L63 L64 L65 L66 L67 L68 L69 L70 L71 L72 L73 L74 L75 L76 L77 L78 L79 L80 L81 L82 L83 L84 L85 L86 L87 L88 L89 L90 L91 L92 L93 L94 L95 L96 L97 L98 L99 L100 L101 L102 L103 L104 L105 L106 L107 L108 L109 L110 L111 L112 L113 L114 L115 L116 L117 L118 L119 L120 L121 L122 L123 L124 L125 L126 L127 L128 L129 L130 L131 L132 L133 L134 L135 L136 L137 L138 L139 L140 L141 L142 L143 L144 L145 L146 L147 L148 L149 L150 L151 L152 L153 L154 L155 L156 L157 L158 L159 L160 L161 L162 L163 L164 L165 L166 L167 L168 L169 L170 L171 L172 L173 L174 L175 L176 L177 L178 L179 L180 L181 L182 L183 L184 L185 L186 L187 L188 L189 L190 L191 L192 L193 L194 L195 L196 L197 L198 L199 L200 L201 L202 L203 L204 L205 L206 L207 L208 L209 L210 L211 L212 L213 L214 L215 L216 L217 L218 L219 L220 L221 L222 L223 L224 L225 L226 L227 L228 L229 L230 L231 L232 L233 L234 L235 L236 L237 L238 L239 L240 L241 L242 L243 L244 L245 L246 L247 L248 L249 L250 L251 L252 L253 L254 L255 L256 L257 L258 L259 L260 L261 L262 L263 L264 L265 L266 L267 L268 L269 L270 L271 L272 L273 L274 L275 L276 L277 L278 L279 L280 L281 L282 L283 L284 L285 L286 L287 L288 L289 L290 L291 L292 L293 L294 L295 L296 L297 L298 L299 L300 L301 L302 L303 L304 L305 L306 L307 L308 L309 L310 L311 L312 L313 L314 L315 L316 L317 L318 L319 L320 L321 L322 L323 L324 L325 L326 L327 L328 L329 L330 L331 L332 L333 L334 L335 L336 L337 L338 L339 L340 L341 L342 L343 L344 L345 L346 L347 L348 L349 L350 L351 L352 L353 L354 L355 L356 L357 L358 L359 L360 L361 L362 L363 L364 L365 L366 L367 L368 L369 L370 L371 L372 L373 L374 L375 L376 L377 L378 L379 L380 L381 L382 L383 L384 L385 L386 L387 L388 L389 L390 L391 L392 L393 L394 L395 L396 L397 L398 L399 L400 L401 L402 L403 L404 L405 L406 L407 L408 L409 L410 L411 L412 L413 L414 L415 L416 L417 L418 L419 L420 L421 L422 L423 L424 L425 L426 L427 L428 L429 L430 L431 L432 L433 L434 L435 L436 L437 L438 L439 L440 L441 L442 L443 L444 L445 L446 L447 L448 L449 L450 L451 L452 L453 L454 L455 L456 L457 L458 L459 L460 L461 L462 L463 L464 L465 L466 L467 L468 L469 L470 L471 L472 L473 L474 L475 L476 L477 L478 L479 L480 L481 L482 L483 L484 L485 L486 L487 L488 L489 L490 L491 L492 L493 L494 L495 L496 L497 L498 L499 L500 L501 L502 L503 L504 L505 L506 L507 L508 L509 L510 L511 L512 L513 L514 L515 L516 L517 L518 L519 L520 L521 L522 L523 L524 L525 L526 L527 L528 L529 L530 L531 L532 L533 L534 L535 L536 L537 L538 L539 L540 L541 L542 L543 L544 L545 L546 L547 L548 L549 L550 L551 L552 L553 L554 L555 L556 L557 L558 L559 L560 L561 L562 L563 L564 L565 L566 L567 L568 L569 L570 L571 L572 L573 L574 L575 L576 L577 L578 L579 L580 L581 L582 L583 L584 L585 L586 L587 L588 L589 L590 L591 L592 L593 L594 L595 L596 L597 L598 L599 L600 L601 L602 L603 L604 L605 L606 L607 L608 L609 L610 L611 L612 L613 L614 L615 L616 L617 L618 L619 L620 L621 L622 L623 L624 L625 L626 L627 L628 L629 L630 L631 L632 L633 L634 L635 L636 L637 L638 L639 L640 L641 L642 L643 L644 L645 L646 L647 L648 L649 L650 L651 L652 L653 L654 L655 L656 L657 L658 L659 L660 L661 L662 L663 L664 L665 L666 L667 L668 L669 L670 L671 L672 L673 L674 L675 L676 L677 L678 L679 L680 L681 L682 L683 L684 L685 L686 L687 L688 L689 L690 L691 L692 L693 L694 L695 L696 L697 L698 L699 L700 L701 L702 L703 L704 L705 L706 L707 L708 L709 L710 L711 L712 L713 L714 L715 L716 L717 L718 L719 L720 L721 L722 L723 L724 L725 L726 L727 L728 L729 L730 L731 L732 L733 L734 L735 L736 L737 L738 L739 L740 L741 L742 L743 L744 L745 L746 L747 L748 L749 L750 L751 L752 L753 L754 L755 L756 L757 L758 L759 L760 L761 L762 L763 L764 L765 L766 L767 L768 L769 L770 L771 L772 L773 L774 L775 L776 L777 L778 L779 L780 L781 L782 L783 L784 L785 L786 L787 L788 L789 L790 L791 L792 L793 L794 L795 L796 L797 L798 L799 L800 L801 L802 L803 L804 L805 L806 L807 L808 L809 L810 L811 L812 L813 L814 L815 L816 L817 L818 L819 L820 L821 L822 L823 L824 L825 L826 L827 L828 L829 L830 L831 L832 L833 L834 L835 L836 L837 L838 L839 L840 L841 L842 L843 L844 L845 L846 L847 L848 L849 L850 L851 L852 L853 L854 L855 L856 L857 L858 L859 L860 L861 L862 L863 L864 L865 L866 L867 L868 L869 L870 L871 L872 L873 L874 L875 L876 L877 L878 L879 L880 L881 L882 L883 L884 L885 L886 L887 L888 L889 L890 L891 L892 L893 L894 L895 L896 L897 L898 L899 L900 L901 L902 L903 L904 L905 L906 L907 L908 L909 L910 L911 L912 L913 L914 L915 L916 L917 L918 L919 L920 L921 L922 L923 L924 L925 L926 L927 L928 L929 L930 L931 L932 L933 L934 L935 L936 L937 L938 L939 L940 L941 L942 L943 L944 L945 L946 L947 L948 L949 L950 L951 L952 L953 L954 L955 L956 L957 L958 L959 L960 L961 L962 L963 L964 L965 L966 L967 L968 L969 L970 L971 L972 L973 L974 L975 L976 L977 L978 L979 L980 L981 L982 L983 L984 L985 L986 L987 L988 L989 L990 L991 L992 L993 L994 L995 L996 L997 L998 L999 L1000 L1001 L1002 L1003 L1004 L1005 L1006 L1007 L1008 L1009 L1010 L1011 L1012 L1013 L1014 L1015 L1016 L1017 L1018 L1019 L1020 L1021 L1022 L1023 L1024 L1025 L1026 L1027 L1028 L1029 L1030 L1031 L1032 L1033 L1034 L1035 L1036 L1037 L1038 L1039 L1040 L1041 L1042 L1043 L1044 L1045 L1046 L1047 L1048 L1049 L1050 L1051 L1052 L1053 L1054 L1055 L1056 L1057 L1058 L1059 L1060 L1061 L1062 L1063 L1064 L1065 L1066 L1067 L1068 L1069 L1070 L1071 L1072 L1073 L1074 L1075 L1076 L1077 L1078 L1079 L1080 L1081 L1082 L1083 L1084 L1085 L1086 L1087 L1088 L1089 L1090 L1091 L1092 L1093 L1094 L1095 L1096 L1097 L1098 L1099 L1100 L1101 L1102 L1103 L1104 L1105 L1106 L1107 L1108 L1109
equation "\"d18\" = Gear_tooth_wall_thickness"
equation "\"d23\" = Gear60_lightener_hole_offset"
equation "\"d24\" = d23"
equation "\"d25\" = d23"
equation "\"d26\" = d25"
equation "\"d27\" = Gear60_lightener_hole_fillet"
equation "\"d32\" = Inner_thickness"
equation "\"Gear60_lightener_hole_offset\" = 2"
equation "\"Gear60_lightener_hole_fillet\" = 2"
equation "\"Gear_tooth_wall_thickness\" = 1"
equation "\"Inner_thickness\" = 1"
body "Solid4"
